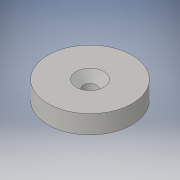
# Autodesk Inventor part: Magnet
Saved by Autodesk Inventor 2016 (Build 200138000, 138)
## iProperties
Created: 2016-07-10
Part Number: Magnet
Material: Generic
Document SubType Name: Modeling
Designer: jeffkub
Density: 1 g/cm^3
Appearance: Default
Author: jeffkub
Autodesk Inventor part; units mm, degrees
ref_plane "YZ Plane" through (0, 0, 0) normal (1, 0, 0) x (0, 1, 0)
ref_plane "XZ Plane" through (0, 0, 0) normal (0, 1, 0) x (-1, 0, 0)
ref_plane "XY Plane" through (0, 0, 0) normal (0, 0, 1) x (1, 0, 0)
sketch "Sketch1" plane through (0, 0, 0) normal (0, 0, 1) x (1, 0, 0)
  line L0 (2.54, 0) -> (2.54, 3.8825)
  line L1 (2.54, 3.8825) -> (5.25, 7)
  line L2 (5.25, 7) -> (16, 7)
  line L3 (16, 7) -> (16, 0)
  line L4 (16, 0) -> (2.54, 0)
  line L5 (0, 14.5655) -> (0, -5.7291)
  point P0 (0, 0)
  dimension "d0" = 5.08
  dimension "d1" = 32
  dimension "d2" = 7
  dimension "d3" = 41
  dimension "d4" = 10.5
  constraints: 12 end point, 3 perpendicular, 2 point on line, 2 vertical
  measures "d0" diameter of L0 L5
  measures "d1" diameter of L3 L5
  measures "d2" distance of L2.end L3.end
  measures "d3" angle of L5 L1
  measures "d4" diameter of L1.end L5
revolve "Revolution1" add sketch "Sketch1" angle 360 about axis through (0, 14.5655, 0) along (0, -1, 0)
body "Solid1"
